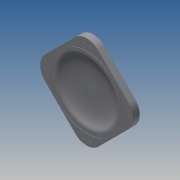
# Autodesk Inventor part: wheel_rim_mold_A
Saved by Autodesk Inventor 2016 (Build 200138000, 138)
## iProperties
Created: 2014-06-11
Part Number: wheel_rim_mold_A
Material: Générique
Document SubType Name: Modeling
Designer: Yann
Density: 1 g/cm^3
Appearance: Par défaut
Mass: 4520.39 g
Surface Area: 4824.92 cm^2
Volume: 4520.39 cm^3
Author: Yann
Autodesk Inventor part; units mm, degrees
ref_plane "YZ Plane" through (0, 0, 0) normal (1, 0, 0) x (0, 1, 0)
ref_plane "XZ Plane" through (0, 0, 0) normal (0, 1, 0) x (-1, 0, 0)
sketch "Esquisse1" plane through (0, 0, 0) normal (0, 1, 0) x (-1, 0, 0)
  circle A0 centre (0, 0) radius 215.2 construction
  line L0 (0, -455.3768) -> (0, 455.3768) projected
  line L1 (-455.3768, 0) -> (455.3768, 0) projected
  line L2 (70.7107, -254.5584) -> (254.5584, -70.7107)
  line L3 (254.5584, 70.7107) -> (70.7107, 254.5584)
  line L4 (-70.7107, 254.5584) -> (-254.5584, 70.7107)
  line L5 (-254.5584, -70.7107) -> (-70.7107, -254.5584)
  line L6 (0, -325.2691) -> (0, 325.2691) construction
  line L7 (325.2691, 0) -> (-325.2691, 0) construction
  circle A1 centre (-20, 253.412) radius 4
  circle A2 centre (11, -19.0526) radius 2.5 projected
  circle A3 centre (-11, -19.0526) radius 2.5 projected
  circle A4 centre (-22, 0) radius 2.5 projected
  circle A5 centre (-11, 19.0526) radius 2.5 projected
  circle A6 centre (11, 19.0526) radius 2.5 projected
  circle A7 centre (22, 0) radius 2.5 projected
  circle A8 centre (0, 0) radius 30 construction
  circle A9 centre (0, 0) radius 13 construction
  arc A10 (-254.5584, 70.7107) -> (-254.5584, -70.7107) centre (-183.8478, 0) ccw
  arc A11 (70.7107, 254.5584) -> (-70.7107, 254.5584) centre (0, 183.8478) ccw
  arc A12 (-70.7107, -254.5584) -> (70.7107, -254.5584) centre (0, -183.8478) ccw
  arc A13 (254.5584, -70.7107) -> (254.5584, 70.7107) centre (183.8478, 0) ccw
  circle A14 centre (20, 253.412) radius 4
  circle A15 centre (-20, -253.412) radius 4
  circle A16 centre (20, -253.412) radius 4
  circle A17 centre (-254.2, 0) radius 4
  circle A18 centre (254.2, 0) radius 4
  point P0 (0, 0)
  dimension "d1" = 460
  dimension "d2" = 8
  dimension "d3" = 35
  dimension "d13" = 100
  dimension "d14" = 20
  dimension "d15" = 35
  constraints: 12 end point, 10 centre point, 9 point on line, 8 point on circle, 8 tangent, 4 equal radius, 4 symmetric about line, 2 midpoint, 2 parallel, 2 perpendicular, 1 horizontal, 4 other
  measures "d1" distance of L6.end L7.start
  measures "d2" diameter of A1
  measures "d13" radius of A10
  measures "d14" distance from line of L6 A1.centre
ref_plane "Plan de construction1" through (-34.1506, 32.18, -34.1506) normal (0, 1, 0) x (0.5, 0, 0.866)
extrude "Extrusion1" add sketch "Esquisse1" along normal blind 40.5 contours A12 L5 A10 L1 A17 A4 L0 | L0 L1 A7 A18 A13 L2 A12 | L1 A4 A17 A10 L4 A11 L0 | L0 A11 L3 A13 L1 A18 A7
sketch "Esquisse2" plane through (0, 0, 0) normal (1, 0, 0) x (0, 1, 0)
  line L0 (0, 215.2) -> (0, -215.2) projected
  spline S0 degree 3 poles (0, 200.2) (0, 197.9965) (0.0414, 194.0177) (0.2008, 189.8631) (0.4177, 186.5163) (0.6028, 184.46) (0.8206, 182.4936) (0.982, 181.2194) (1.2042, 179.6533) (1.3983, 178.4142) (1.6613, 176.8647) (1.888, 175.618) (2.1914, 174.0353) (2.4501, 172.7437) (2.7925, 171.0841) (3.0815, 169.7154) (3.4603, 167.9416) (3.7771, 166.468) (4.1888, 164.5477) (4.5301, 162.9452) (4.9701, 160.8505) (5.3322, 159.0985) (5.7956, 156.8056) (6.1744, 154.8864) (6.6558, 152.3752) (7.0467, 150.2743) (7.5403, 147.5283) (7.9384, 145.2341) (8.4378, 142.2409) (8.838, 139.7448) (9.3365, 136.4958) (9.7331, 133.7934) (10.2239, 130.2876) (10.6118, 127.3818) (11.0888, 123.6275) (11.4634, 120.5287) (11.9212, 116.5436) (12.2783, 113.2699) (12.712, 109.0815) (13.0481, 105.6586) (13.4534, 101.3039) (13.7653, 97.7655) (14.1386, 93.2913) (14.4236, 89.6786) (14.7619, 85.1416) (15.0179, 81.5039) (15.3187, 76.9704) (15.5438, 73.3647) (15.8053, 68.9108) (15.9983, 65.4019) (16.2191, 61.1136) (16.3793, 57.7741) (16.5587, 53.7471) (16.6856, 50.6574) (16.8236, 46.997) (16.9174, 44.2452) (17.0143, 41.066) (17.0757, 38.7475) (17.127, 36.4302) (17.1514, 35.0579) (17.1682, 33.8363) (17.1775, 32.9151) (17.18, 32.2864) (17.18, 32) knots 1 1 1 1 1.083333 1.166667 1.208333 1.270833 1.291667 1.333333 1.354167 1.395833 1.416667 1.458333 1.479167 1.520833 1.541667 1.583333 1.604167 1.645833 1.666667 1.708333 1.729167 1.770833 1.791667 1.833333 1.854167 1.895833 1.916667 1.958333 1.979167 2.020833 2.041667 2.083333 2.104167 2.145833 2.166667 2.208333 2.229167 2.270833 2.291667 2.333333 2.354167 2.395833 2.416667 2.458333 2.479167 2.520833 2.541667 2.583333 2.604167 2.645833 2.666667 2.708333 2.729167 2.770833 2.791667 2.833333 2.854167 2.895833 2.916667 2.947917 2.958333 2.979167 3 3 3 3 projected
  line L1 (17.18, 32) -> (17.18, -32) projected
  line L2 (17.18, 0) -> (0, 0)
  line L3 (-6.6319, 0) -> (26.4905, 0) projected
  line L4 (0, 215.2) -> (2, 215.2)
  line L5 (2, 215.2) -> (2, 220.2)
  line L6 (2, 220.2) -> (0, 220.2)
  line L7 (0, 220.2) -> (0, 215.2)
  point P0 (0, 200.2)
  dimension "d11" = 5
  dimension "d12" = 2
  constraints: 10 end point, 3 parallel, 2 midpoint, 2 perpendicular, 1 point on line, 1 other
  measures "d11" distance of L6.end L0.start
  measures "d12" distance of L0.start L4.end
revolve "Révolution1" cut sketch "Esquisse2" angle 360 about axis through (0, -10, 0) along (0, 1, 0)
equation "\"d15\" = d3"
